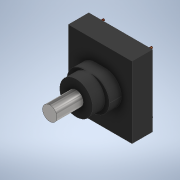
# Autodesk Inventor part: Encoder
Saved by Autodesk Inventor 2020 (Build 240168000, 168)
## iProperties
Created: 2021-07-01
Part Number: Encoder
Material: ABS Plastic
Document SubType Name: Modeling
Designer: 10300812
Density: 1.06 g/cm^3
Appearance: Rubber - Black
Author: 10300812
Autodesk Inventor part; units mm, degrees
ref_plane "YZ Plane" through (0, 0, 0) normal (1, 0, 0) x (0, 1, 0)
ref_plane "XZ Plane" through (0, 0, 0) normal (0, 1, 0) x (-1, 0, 0)
ref_plane "XY Plane" through (0, 0, 0) normal (0, 0, 1) x (1, 0, 0)
sketch "Sketch1" plane through (0, 0, 0) normal (0, 0, 1) x (1, 0, 0)
  line L0 (-13.25, 14.85) -> (13.25, 14.85)
  line L1 (13.25, 14.85) -> (13.25, -14.85)
  line L2 (13.25, -14.85) -> (-13.25, -14.85)
  line L3 (-13.25, -14.85) -> (-13.25, 14.85)
  line L4 (-13.25, 14.85) -> (13.25, -14.85) construction
  line L5 (13.25, 14.85) -> (-13.25, -14.85) construction
  point P0 (0, 0)
  dimension "d0" = 26.5
  dimension "d1" = 29.7
  constraints: 12 end point, 2 midpoint, 2 parallel, 1 horizontal, 1 perpendicular
  measures "d0" distance of L1.end L2.end
  measures "d1" distance of L0.end L1.end
extrude "Extrusion1" add sketch "Sketch1" along normal blind 8.5
sketch "Sketch2" plane through (0, 0, 8.5) normal (0, 0, 1) x (1, 0, 0)
  line L0 (-8.8, 6.85) -> (8.8, 6.85)
  line L1 (8.8, 6.85) -> (8.8, -6.85)
  line L2 (8.8, -6.85) -> (-8.8, -6.85)
  line L3 (-8.8, -6.85) -> (-8.8, 6.85)
  line L4 (-8.8, 6.85) -> (8.8, -6.85) construction
  line L5 (8.8, 6.85) -> (-8.8, -6.85) construction
  point P0 (0, 0)
  dimension "d4" = 17.6
  dimension "d5" = 13.7
  constraints: 12 end point, 2 midpoint, 2 parallel, 1 horizontal, 1 perpendicular
  measures "d4" distance of L1.end L2.end
  measures "d5" distance of L0.end L1.end
extrude "Extrusion2" add sketch "Sketch2" along normal blind 5
fillet "Fillet1" radius 6.8 4 edges at (8.8, 6.85, 11) (8.8, -6.85, 11) (-8.8, 6.85, 11) (-8.8, -6.85, 11)
sketch "Sketch3" plane through (0, 0, 13.5) normal (0, 0, 1) x (1, 0, 0)
  circle A0 centre (0, 0) radius 6.825
  dimension "d9" = 13.65
  constraints: 1 centre point, 1 coincident
  measures "d9" diameter of A0
extrude "Extrusion3" add sketch "Sketch3" along normal blind 5
sketch "Sketch4" plane through (0, 0, 18.5) normal (0, 0, 1) x (1, 0, 0)
  circle A0 centre (0, 0) radius 3
  dimension "d12" = 6
  constraints: 1 centre point, 1 coincident
  measures "d12" diameter of A0
extrude "Extrusion4" add sketch "Sketch4" along normal blind 11
sketch "Sketch5" plane through (0, 0, 0) normal (0, 0, -1) x (-1, 0, 0)
  line L0 (-10, 12.5) -> (10, 12.5) construction
  line L1 (10, 12.5) -> (10, -12.5) construction
  line L2 (10, -12.5) -> (-10, -12.5) construction
  line L3 (-10, -12.5) -> (-10, 12.5) construction
  line L4 (-10, 12.5) -> (10, -12.5) construction
  line L5 (10, 12.5) -> (-10, -12.5) construction
  circle A0 centre (10, 12.5) radius 0.4
  circle A1 centre (-10, -12.5) radius 0.4
  circle A2 centre (10, -12.5) radius 0.4
  circle A3 centre (-10, 12.5) radius 0.4
  point P0 (0, 0)
  dimension "d15" = 20
  dimension "d16" = 25
  dimension "d18" = 0.8
  dimension "d19" = 0.8
  dimension "d20" = 0.8
  dimension "d21" = 0.8
  constraints: 12 end point, 4 centre point, 4 coincident, 2 midpoint, 2 parallel, 1 horizontal, 1 perpendicular
  measures "d15" distance of L1.end L2.end
  measures "d16" distance of L0.end L1.end
  measures "d18" diameter of A0
  measures "d19" diameter of A1
  measures "d20" diameter of A2
  measures "d21" diameter of A3
extrude "Extrusion5" add sketch "Sketch5" along normal blind 3
sketch "Sketch6" plane through (0, 0, 0) normal (0, 0, -1) x (-1, 0, 0)
  circle A0 centre (0, 0) radius 6.825 projected
extrude "Extrusion6" add sketch "Sketch6" along normal blind 4
body "Solid1"
